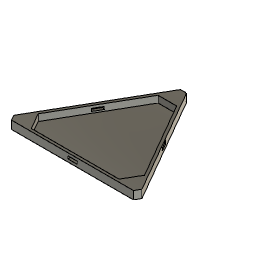
Vriksha (Nanoleaf) (Autodesk Fusion 360 design; units mm, degrees)
Autodesk Fusion 360 part; units mm, degrees
sketch "Sketch1" plane through (0, 0, 0) normal (0, 0, 1) x (1, 0, 0) in component "base"
  line L0 (0, 0) -> (0, 216.506)
  line L1 (0, 216.506) -> (125, -0.0004)
  line L2 (125, -0.0004) -> (-125, -0.0004)
  line L3 (-125, -0.0004) -> (0, 216.506)
  dimension "d7" = 216.506
  dimension "d8" = 30
  dimension "d9" = 250
  dimension "d10" = 250
  constraint vertical L0
  constraint coincident L0.start origin
  constraint horizontal L2
  measures "d7" distance of L0.start L0.end
  measures "d8" angle of L0 L1
  measures "d9" distance of L0.end L1.end
  measures "d10" distance of L1.end L2.end
extrude "Extrude1" add sketch "Sketch1" along normal blind 15 makes body 1 in component "base"
split "Split1" by plane through (0, 206.506, 7.5) normal (0, 1, 0) bodies 1 makes body 2 at (1.9245, 213.1727, 5) in component "base"
split "Split2" by plane through (-116.3397, 4.9996, 7.5) normal (-0.866025, -0.5, 0) bodies 1 makes body 3 at (-121.151, 6.6663, 5) in component "base"
split "Split3" by plane through (116.3397, 4.9996, 7.5) normal (-0.866025, 0.5, 0) bodies 1 makes body 4 at (-41.6667, 72.1684, 0) in component "base"
ref_plane "WorkPlane7" through (90.359, 19.9996, 7.5) normal (0.866025, -0.5, 0) x (0, 0, -1) in component "base"
ref_plane "WorkPlane8" through (0, 176.506, 7.5) normal (0, 1, 0) x (0, 0, 1) in component "base"
ref_plane "WorkPlane9" through (-90.359, 19.9996, 7.5) normal (-0.866025, -0.5, 0) x (0, 0, 1) in component "base"
ref_plane "WorkPlane10" through (0, 4.9996, 7.5) normal (0, -1, 0) x (1, 0, 0) in component "base"
ref_plane "WorkPlane11" through (58.1699, 105.7528, 7.5) normal (0.866025, 0.5, 0) x (-0.5, 0.866025, 0) in component "base"
ref_plane "WorkPlane12" through (-58.1699, 105.7528, 7.5) normal (-0.866025, 0.5, 0) x (-0.5, -0.866025, 0) in component "base"
split "Split4" by plane through (-90.359, 19.9996, 7.5) normal (-0.866025, -0.5, 0) bodies 4 makes body 5 at (-98.057, 13.333, 0) in component "base"
split "Split5" by plane through (0, 4.9996, 7.5) normal (0, -1, 0) bodies 4 makes body 6 at (75.6353, -0.0004, 5) in component "base"
split "Split6" by plane through (90.359, 19.9996, 7.5) normal (0.866025, -0.5, 0) bodies 4 makes body 7 at (100.9437, 18.333, 0) in component "base"
split "Split7" by plane through (-58.1699, 105.7528, 7.5) normal (-0.866025, 0.5, 0) bodies 4 makes body 8 at (-69.8618, 95.5018, 10) in component "base"
split "Split8" by plane through (0, 176.506, 7.5) normal (0, 1, 0) bodies 4 makes body 9 at (3.849, 186.506, 0) in component "base"
split "Split9" by plane through (58.1699, 105.7528, 7.5) normal (0.866025, 0.5, 0) bodies 4 makes body 10 at (49.3647, 131.0039, 5) in component "base"
combine "Combine1" operation add target body 5 tool bodies 6 7 10 9 8 in component "base"
extrude "Extrude2" cut 1 faces at (0, 72.1684, 15) along direction (0, 0, -1) blind 12.5 on bodies 4 bodies 4 in component "base"
box "BoxPrimitive1" add length 10 width 10 height 8 placed x (0, -1, 0) y (1, 0, 0) z (0, 0, 1) at (-170.1181, 136.492, 2.5) separate body makes body 11 in component "base"
move_body "Move1" bodies 11 to x (1, 0, 0) y (0, 1, 0) z (0, 0, 1) at (165, 0, 1) in component "base"
move_body "Move2" bodies 11 to x (1, 0, 0) y (0, 1, 0) z (0, 0, 1) at (0, -128, 0) in component "base"
copy_body "CopyPasteBodies1" bodies 11 makes body 12 in component "base"
move_body "Move3" bodies 12 to x (0.5, -0.866025, 0) y (0.866025, 0.5, 0) z (0, 0, 1) at (55.5904, 108.1536, -0.0962) in component "base"
move_body "Move4" bodies 12 to x (1, 0, 0) y (0, 1, 0) z (0, 0, 1) at (2.7479, -0.9016, -0.3102) in component "base"
move_body "Move5" bodies 12 to x (1, 0, 0) y (0, 1, 0) z (0, 0, 1) at (0, 108.253, 0) in component "base"
move_body "Move6" bodies 12 to x (1, 0, 0) y (0, 1, 0) z (0, 0, 1) at (62.5, 108.253, 7.5) in component "base"
move_body "Move7" bodies 12 to x (1, 0, 0) y (0, 1, 0) z (0, 0, 1) at (62.5, 108.253, 7.5) in component "base"
move_body "Move8" bodies 12 to x (1, 0, 0) y (0, 1, 0) z (0, 0, 1) at (-131.1155, -315.7685, -8.6908) in component "base"
move_body "Move9" bodies 12 to x (1, 0, 0) y (0, 1, 0) z (0, 0, 1) at (0, 0, -5) in component "base"
move_body "Move10" bodies 12 to x (1, 0, 0) y (0, 1, 0) z (0, 0, 1) at (5.3821, -10.654, -1.0894) in component "base"
copy_body "CopyPasteBodies2" bodies 12 makes body 13 in component "base"
move_body "Move11" bodies 13 to x (0.866025, 0.5, 0) y (-0.5, 0.866025, 0) z (0, 0, 1) at (-60.0257, -21.3816, 1.5491) in component "base"
move_body "Move12" bodies 13 to x (1, 0, 0) y (0, 1, 0) z (0, 0, 1) at (0, 3.0456, -0.9967) in component "base"
move_body "Move13" bodies 13 to x (1, 0, 0) y (0, 1, 0) z (0, 0, 1) at (0, 2.1754, 0.1034) in component "base"
move_body "Move14" bodies 12 to x (1, 0, 0) y (0, 1, 0) z (0, 0, 1) at (0, -0.6591, 0.3593) in component "base"
move_body "Move15" bodies 12 to x (1, 0, 0) y (0, 1, 0) z (0, 0, 1) at (0, 0.4394, 0.3928) in component "base"
combine "Combine2" operation cut target body 5 tool bodies 13 in component "base"
combine "Combine3" operation cut target body 5 tool bodies 11 in component "base"
combine "Combine4" operation cut target body 5 tool bodies 12 in component "base"
combine "Combine5" operation add target body 5 tool bodies 4 in component "base"
extrude "Extrude3" cut 1 faces at (-5.1181, 3.333, 6.1667) along direction (-1, 0, 0) blind 2 on bodies 5 bodies 5 in component "base"
extrude "Extrude4" cut 1 faces at (4.8819, 1.6663, 6.1667) along direction (1, 0, 0) blind 2 on bodies 5 bodies 5 in component "base"
extrude "Extrude5" cut 1 faces at (-7.1181, 3.333, 6.1667) along direction (-1, 0, 0) blind 1.5 on bodies 5 bodies 5 in component "base"
extrude "Extrude6" cut 1 faces at (6.8819, 1.6663, 6.1667) along direction (1, 0, 0) blind 1.5 on bodies 5 bodies 5 in component "base"
extrude "Extrude7" add 1 faces at (-2.9514, 3.333, 3.5) along direction (0, 0, 1) blind 1.5 on bodies 5 bodies 5 in component "base"
extrude "Extrude8" add 1 faces at (2.7153, 1.6663, 11.5) along direction (0, 0, -1) blind 1.5 on bodies 5 bodies 5 in component "base"
extrude "Extrude9" cut 1 faces at (-58.7239, 111.46, 6.6359) along direction (0.5, 0.866025, 0) blind 3.5 on bodies 5 bodies 5 in component "base"
extrude "Extrude10" cut 1 faces at (-63.7239, 102.7997, 6.6359) along direction (-0.5, -0.866025, 0) blind 3.5 on bodies 5 bodies 5 in component "base"
extrude "Extrude11" add 1 faces at (-59.8072, 109.5836, 3.9692) along direction (0, 0, 1) blind 1.5 on bodies 5 bodies 5 in component "base"
extrude "Extrude12" add 1 faces at (-59.8072, 109.5836, 11.9692) along direction (0, 0, -1) blind 1.5 on bodies 5 bodies 5 in component "base"
extrude "Extrude13" cut 1 faces at (63.5226, 103.1482, 6.7322) along direction (0.5, -0.866025, 0) blind 3.5 on bodies 5 bodies 5 in component "base"
extrude "Extrude14" add 1 faces at (60.7726, 107.9114, 4.0655) along direction (0, 0, 1) blind 1.5 on bodies 5 bodies 5 in component "base"
extrude "Extrude15" add 1 faces at (60.7726, 107.9114, 12.0655) along direction (0, 0, -1) blind 1.5 on bodies 5 bodies 5 in component "base"
extrude "Extrude16" cut 1 faces at (58.5226, 111.8085, 7.2322) along direction (-0.5, 0.866025, 0) blind 3.5 on bodies 5 bodies 5 in component "base"
component "base" placed x (1, 0, 0) y (0, 1, 0) z (0, 0, 1) at (0, 0, 0)
hidden bodies 1 2 3
